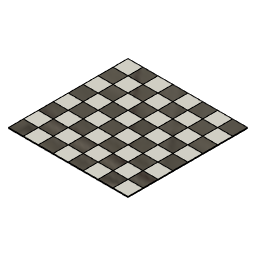
Chessboard 2 v2 (Autodesk Fusion 360 design; units mm, degrees)
Autodesk Fusion 360 part; units mm, degrees
sketch "Sketch1" plane through (0, 0, 0) normal (0, 0, 1) x (1, 0, 0) in component "Square"
  line L0 (0, 0) -> (100, 0)
  line L1 (100, 0) -> (100, 100)
  line L2 (100, 100) -> (0, 100)
  line L3 (0, 100) -> (0, 0)
  line L4 (100, 100) -> (200, 100)
  line L5 (200, 100) -> (200, 200)
  line L6 (200, 200) -> (100, 200)
  line L7 (100, 200) -> (100, 100)
  dimension "d1" = 100
  dimension "d2" = 100
  dimension "d3" = 100
  dimension "d4" = 100
  constraint horizontal L0
  constraint vertical L1
  constraint horizontal L2
  constraint vertical L3
  constraint coincident L0.start L3.end
  constraint horizontal L4
  constraint vertical L5
  constraint horizontal L6
  constraint vertical L7
  measures "d1" distance of L0.start L0.end
  measures "d2" distance of L0.start L2.end
  measures "d3" distance of L1.end L4.end
  measures "d4" distance of L1.end L6.end
extrude "Extrude1" add sketch "Sketch1" along normal blind 5 makes body 1 in component "Square"
pattern_linear "R-Pattern1" count 4 spacing 200 along (0, -1, 0) count 4 spacing 200 along (1, 0, 0) of bodies 1 makes body 2 at (33.3333, -133.3333, 0) makes body 3 at (33.3333, -333.3333, 0) makes body 4 at (33.3333, -533.3333, 0) makes body 5 at (233.3333, 66.6667, 0) makes body 6 at (233.3333, -133.3333, 0) makes body 7 at (233.3333, -333.3333, 0) makes body 8 at (233.3333, -533.3333, 0) makes body 9 at (433.3333, 66.6667, 0) makes body 10 at (433.3333, -133.3333, 0) makes body 11 at (433.3333, -333.3333, 0) makes body 12 at (433.3333, -533.3333, 0) makes body 13 at (633.3333, 66.6667, 0) makes body 14 at (633.3333, -133.3333, 0) makes body 15 at (633.3333, -333.3333, 0) makes body 16 at (633.3333, -533.3333, 0) in component "Square"
combine "Combine1" operation add target body 1 tool bodies 2 3 4 5 6 7 8 9 10 11 12 13 14 15 16 in component "Square"
move_body "Move1" bodies 1 to x (0, 1, 0) y (-1, 0, 0) z (0, 0, 1) at (200, -600, 0) in component "Square"
copy_body "CopyPasteBodies1" bodies 1 makes body 17 in component "Square"
move_body "Move2" bodies 17 to x (0, 1, 0) y (-1, 0, 0) z (0, 0, 1) at (200, -600, 0) in component "Square"
move_body "Move3" bodies 17 to x (1, 0, 0) y (0, 1, 0) z (0, 0, 1) at (841.7371, 0, 9.7971) in component "Square"
scale "Scale1" factor 0.43 about (941.7371, 200, 14.7971) bodies 17 in component "Square"
scale "Scale2" factor 0.43 about (0, -100, 5) bodies 1 in component "Square"
move_body "Move4" bodies 1 to x (1, 0, 0) y (0, 1, 0) z (0, 0, 1) at (396.9489, 285.1473, -111.8016) in component "Square"
move_body "Move5" bodies 1 to x (1, 0, 0) y (0, 1, 0) z (0, 0, 1) at (251.6079, 129.6383, -121.9696) in component "Square"
move_body "Move6" bodies 1 to x (1, 0, 0) y (0, 1, 0) z (0, 0, 1) at (6, 0, 0) in component "Square"
move_body "Move7" bodies 1 to x (1, 0, 0) y (0, 1, 0) z (0, 0, 1) at (244.1803, -243.7856, 243.5682) in component "Square"
component "Square" placed x (1, 0, 0) y (0, 1, 0) z (0, 0, 1) at (0, 0, 0)
